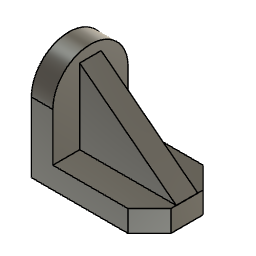
A1 (Autodesk Fusion 360 design; units mm, degrees)
Autodesk Fusion 360 part; units mm, degrees
sketch "Baza" plane through (0, 0, 0) normal (0, 0, 1) x (1, 0, 0)
  line L0 (33, 21) -> (-33, 21)
  line L1 (-33, 21) -> (-33, -21)
  line L2 (-33, -21) -> (33, -21)
  line L3 (33, -21) -> (33, 21)
  line L4 (33, 21) -> (-33, -21) construction
  line L5 (-33, 21) -> (33, -21) construction
  dimension "d1" = 42
  dimension "d2" = 66
  constraint horizontal L0
  constraint perpendicular L0 L1
  constraint parallel L0 L2
  constraint parallel L1 L3
  constraint coincident L4 origin
  constraint coincident L5 origin
  measures "d1" distance of L0.end L1.end
  measures "d2" distance of L0.start L0.end
extrude "Extrude1" add sketch "Baza" along normal blind 12
chamfer "Chamfer1" distance 12 angle 45 2 edges at (33, -21, 6) (33, 21, 6)
sketch "Baza 2" plane through (0, 0, 12) normal (0, 0, 1) x (-1, 0, 0)
  line L0 (-33, -9) -> (-21, -21)
  line L1 (-21, -21) -> (33, -21)
  line L2 (33, -21) -> (33, 21)
  line L3 (33, 21) -> (-21, 21)
  line L4 (-21, 21) -> (-33, 9)
  line L5 (-33, 9) -> (-33, -9)
  line L6 (33, -21) -> (21, -21)
  line L7 (21, -21) -> (21, 21)
  line L8 (21, 21) -> (33, 21)
  line L9 (33, 21) -> (33, -21)
  dimension "d9" = 12
  constraint horizontal L6
  constraint vertical L7
  constraint horizontal L8
  constraint vertical L9
  constraint coincident L1.end L2.start
  measures "d9" distance of L1.end L6.end
extrude "Extrude3" add sketch "Baza 2" along normal blind 48 contours L1 L2 L3 L6 L7 L8 L9
fillet "Fillet1" radius 21 2 edges at (-27, -21, 60) (-27, 21, 60)
sketch "Triunghi" plane through (0, 0, 0) normal (0, 1, 0) x (1, 0, 0)
  line L0 (-20.989, -53.9545) -> (-20.989, -11.9545)
  line L1 (-20.989, -11.9545) -> (33.011, -11.9545)
  line L2 (33.011, -11.9545) -> (-20.989, -53.9545)
  dimension "d14" = 42
  dimension "d15" = 54
  constraint vertical L0
  constraint perpendicular L0 L1
  measures "d14" distance of L0.start L0.end
  measures "d15" distance of L0.end L1.end
extrude "Extrude4" add sketch "Triunghi" along normal mid plane 12
sketch "Nu apasa" plane through (-33, 0, 0) normal (-1, 0, 0) x (0, -1, 0)
  arc A0 (21, 39) -> (-21, 39) centre (0, 39) ccw
  line L0 (-21, 39) -> (-21, 0)
  line L1 (-21, 0) -> (21, 0)
  line L2 (21, 0) -> (21, 39)
  line L3 (-8.5043, 34.4587) -> (8.0682, 34.4186) construction
  line L4 (8.0682, 34.4186) -> (8.0781, 38.5306) construction
  line L5 (8.0781, 38.5306) -> (-8.4944, 38.5707) construction
  line L6 (-8.4944, 38.5707) -> (-8.5043, 34.4587) construction
equation "d10 = 60 mm - 12 mm"
equation "d15 = 66 mm - 12 mm"
named bodies: "A1"
